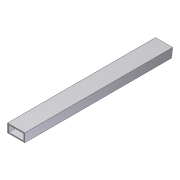
# Autodesk Inventor part: FE-00013-05
Saved by Autodesk Inventor 2012 (Build 160160000, 160)
## iProperties
Created: 2008-05-28
Part Number: FE-00013-05
Description: Support
Document SubType Name: Modeling
Designer: narosenberg
Density: 1 g/cm^3
Mass: 192.955 g
Surface Area: 1224.38 cm^2
Volume: 192.955 cm^3
Material: Default
Author: narosenberg
Autodesk Inventor part; units mm, degrees
ref_plane "YZ Plane" through (0, 0, 0) normal (1, 0, 0) x (0, 1, 0)
ref_plane "XZ Plane" through (0, 0, 0) normal (0, 1, 0) x (-1, 0, 0)
ref_plane "XY Plane" through (0, 0, 0) normal (0, 0, 1) x (1, 0, 0)
sketch "Sketch1" plane through (0, 0, 0) normal (0, 0, 1) x (1, 0, 0)
  line L0 (-21.7703, 20.0792) -> (29.0297, 20.0792)
  line L1 (29.0297, 20.0792) -> (29.0297, -5.3208)
  line L2 (29.0297, -5.3208) -> (-21.7703, -5.3208)
  line L3 (-21.7703, -5.3208) -> (-21.7703, 20.0792)
  dimension "d0" = 25.4
  dimension "d1" = 50.8
  constraints: 8 end point, 2 parallel, 1 horizontal, 1 perpendicular
  measures "d0" distance of L0.end L1.end
  measures "d1" distance of L0.start L0.end
extrude "Extrusion1" add sketch "Sketch1" along normal blind 436.88
shell "Shell1" thickness 3.175 removed faces 2 at (-4.8369, 11.6125, 436.88) at (-4.8369, 11.6125, 0)
draft "FaceDraft1" angle 8.3 pull direction (0, -1, 0) faces at (-3.7786, 19.0209, 0) fixed edges at (3.6297, 20.0792, 0)
body "Solid1"
